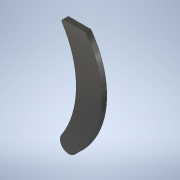
# Autodesk Inventor part: Part40
Saved by Autodesk Inventor 2021 (Build 250183000, 183)
## iProperties
Created: 2020-11-16
Part Number: Part40
Material: Liga de Nickel-Copper 400
Document SubType Name: Modeling
Designer: Lucas Moura
Density: 8.83 g/cm^3
Appearance: Cromado - Preto polido
Author: Lucas Moura
Autodesk Inventor part; units mm, degrees
ref_plane "YZ Plane" through (0, 0, 0) normal (1, 0, 0) x (0, 1, 0)
ref_plane "XZ Plane" through (0, 0, 0) normal (0, 1, 0) x (-1, 0, 0)
ref_plane "XY Plane" through (0, 0, 0) normal (0, 0, 1) x (1, 0, 0)
sketch "Sketch1" plane through (0, 0, 0) normal (0, 0, 1) x (1, 0, 0)
  arc A0 (11.4498, 7.2597) -> (11.1125, 26.7625) centre (-3.0917, 16.7625) ccw
  arc A1 (11.4498, 7.2597) -> (13.9324, 5.1544) centre (12.8228, 6.3624) ccw
  arc A2 (13.9324, 5.1544) -> (16.1125, 26.7625) centre (2.8844, 17.1831) ccw
  line L0 (11.1125, 26.7625) -> (16.1125, 26.7625)
  point P0 (0, 0)
  constraints: 6 point on circle, 3 centre point, 2 end point, 2 tangent, 1 horizontal
extrude "Extrusion1" add sketch "Sketch1" along normal blind 1
sketch "Sketch2" plane through (0, 0, 1) normal (0, 0, 1) x (1, 0, 0)
  arc A0 (11.4498, 7.2597) -> (11.1125, 26.7625) centre (-3.0917, 16.7625) ccw projected
  arc A1 (11.4498, 7.2597) -> (13.9324, 5.1544) centre (12.8228, 6.3624) ccw projected
  arc A2 (13.9324, 5.1544) -> (16.1125, 26.7625) centre (2.8844, 17.1831) ccw projected
  line L0 (16.1125, 26.7625) -> (11.1125, 26.7625) projected
  circle A3 centre (12.8228, 6.3624) radius 0.75
  point P0 (0, 0)
  dimension "d5" = 1.5
  constraints: 1 centre point, 1 coincident
  measures "d5" diameter of A3
extrude "Extrusion2" add sketch "Sketch2" against normal blind 3.5 contours A3
fillet "Fillet1" radius 0.4 1 edges at (11.1125, 26.7625, 0.5)
body "Solid1"
